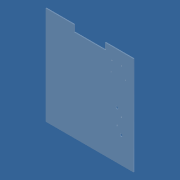
# Autodesk Inventor part: top plate
Saved by Autodesk Inventor 2012 (Build 160160000, 160)
## iProperties
Created: 2012-03-16
Part Number: top plate
Material: Polycarbonate, Clear
Document SubType Name: Modeling
Designer: Ed
Mass: 2419.06 g
Surface Area: 6511.83 cm^2
Volume: 2015.88 cm^3
Density: 1.2 g/cm^3
Author: Ed
Autodesk Inventor part; units mm, degrees
ref_plane "YZ Plane" through (0, 0, 0) normal (1, 0, 0) x (0, 1, 0)
ref_plane "XZ Plane" through (0, 0, 0) normal (0, 1, 0) x (-1, 0, 0)
ref_plane "XY Plane" through (0, 0, 0) normal (0, 0, 1) x (1, 0, 0)
sketch "Sketch1" plane through (0, 0, 0) normal (0, 0, 1) x (1, 0, 0)
  line L0 (0, 0) -> (539.75, 0)
  line L1 (539.75, 0) -> (539.75, 603.25)
  line L2 (539.75, 603.25) -> (0, 603.25)
  line L3 (0, 603.25) -> (0, 0)
  line L4 (174.625, 603.25) -> (365.125, 603.25)
  line L5 (365.125, 603.25) -> (365.125, 563.25)
  line L6 (365.125, 563.25) -> (174.625, 563.25)
  line L7 (174.625, 563.25) -> (174.625, 603.25)
  point P0 (269.875, 603.25)
  dimension "d0" = 603.25
  dimension "d1" = 539.75
  dimension "d4" = 40
  dimension "d5" = 190.5
  constraints: 16 end point, 4 parallel, 2 horizontal, 2 midpoint, 2 perpendicular, 1 point on line
  measures "d0" distance of L2.end L0.start
  measures "d1" distance of L0.start L0.end
  measures "d4" distance of L4.end L5.end
  measures "d5" distance of L5.end L6.end
extrude "Extrusion1" add sketch "Sketch1" along normal blind 6.35 contours L3 L2 L7 L6 L5 L1 L0
hole "Hole1" at (463.55, 527.05, 0) direction (0, 0, 1) diameter 4.4958 end through all clearance for "Flat Head Machine Screw (82)" size "#8" standard "Ansi Unified Screw Threads"
hole "Hole2" at (404.876, 527.05, 0) direction (0, 0, 1) diameter 4.4958 end through all clearance for "Flat Head Machine Screw (82)" size "#8" standard "Ansi Unified Screw Threads"
sketch "Sketch2" plane through (0, 0, 0) normal (0, 0, -1) x (-1, 0, 0)
  line L0 (-539.75, 603.25) -> (-365.125, 603.25) projected
  line L1 (-539.75, 0) -> (-539.75, 603.25) projected
  line L2 (-174.625, 563.25) -> (-365.125, 563.25) projected
  line L3 (-488.95, 463.55) -> (-400.05, 463.55)
  point P0 (-444.5, 463.55)
  dimension "d24" = 88.9
  dimension "d25" = 50.8
  dimension "d27" = 139.7
  constraints: 2 end point, 1 midpoint, 1 parallel
  measures "d24" distance of L3.start L3.end
  measures "d25" distance from line of L1 L3.start
  measures "d27" distance between parallel lines of L0 L3
hole "Hole3" at (488.95, 463.55, 0) at (400.05, 463.55, 0) direction (0, 0, 1) diameter 3.81 end through all clearance for "Flat Head Machine Screw (82)" size "#6" standard "Ansi Unified Screw Threads"
hole "Hole4" at (463.55, 254, 0) direction (0, 0, 1) diameter 6.7564 end through all clearance for "Flat Head Machine Screw (82)" size "1/4" standard "Ansi Unified Screw Threads"
hole "Hole5" at (436.88, 197.358, 0) direction (0, 0, 1) diameter 6.7564 end through all clearance for "Flat Head Machine Screw (82)" size "1/4" standard "Ansi Unified Screw Threads"
sketch "Sketch3" plane through (0, 0, 0) normal (0, 0, -1) x (-1, 0, 0)
  circle A0 centre (-436.88, 197.358) radius 3.3782 projected
  circle A1 centre (-463.55, 254) radius 3.3782 projected
  point P0 (-436.88, 292.1)
  point P1 (-463.55, 158.75)
  dimension "d53" = 133.35
  dimension "d54" = 38.1
  constraints: 2 vertical alignment
  measures "d53" vertical distance of point (-436.88, 292.1) point (-463.55, 158.75)
  measures "d54" vertical distance of point (-436.88, 292.1) A1.centre
hole "Hole6" at (436.88, 292.1, 0) at (463.55, 158.75, 0) direction (0, 0, 1) diameter 15.875 end through all
body "Solid1"
